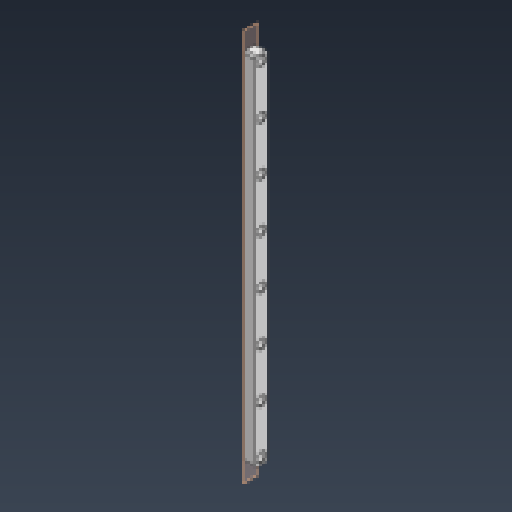
# Autodesk Inventor part: petg_holder
Saved by Autodesk Inventor 2023 (Build 270158000, 158)
## iProperties
Created: 2026-01-24
Part Number: petg_holder
Material: Generic
Document SubType Name: Modeling
Designer: szymo
Density: 1 g/cm^3
Appearance: Default
Author: szymo
Autodesk Inventor part; units mm, degrees
ref_plane "YZ Plane" through (0, 0, 0) normal (1, 0, 0) x (0, 1, 0)
ref_plane "XZ Plane" through (0, 0, 0) normal (0, 1, 0) x (-1, 0, 0)
ref_plane "XY Plane" through (0, 0, 0) normal (0, 0, 1) x (1, 0, 0)
ref_plane "Work Plane1" through (-122.5, -83, 0) normal (1, 0, 0) x (0, -1, 0)
sketch "Sketch1" plane through (-122.5, -83, 0) normal (1, 0, 0) x (0, -1, 0)
  circle A0 centre (-140.1429, -3) radius 1.8 projected
  circle A1 centre (-94.4286, -3) radius 1.8 projected
  circle A2 centre (-48.7143, -3) radius 1.8 projected
  circle A3 centre (-3, -3) radius 1.8 projected
  circle A4 centre (-25.8571, -3) radius 1.8 projected
  circle A5 centre (-71.5714, -3) radius 1.8 projected
  circle A6 centre (-117.2857, -3) radius 1.8 projected
  circle A7 centre (-163, -3) radius 1.8 projected
  line L0 (-166, -6) -> (0, -6) projected
  line L1 (0, 0) -> (0, -6) projected
  line L2 (-166, 0) -> (0, 0) projected
  line L3 (-166, -6) -> (-166, 0) projected
  point P0 (-83, 0)
extrude "Extrusion1" add sketch "Sketch1" along normal blind 5
fillet "Fillet1" radius 1 4 edges at (-120, -83, 0) (-120, -83, 6) (-120, 83, 6) (-120, 83, 0)
sketch "Sketch2" plane through (-117.5, -83, 0) normal (1, 0, 0) x (0, 0, -1)
  arc A0 (0, 165) -> (-1, 166) centre (-1, 165) ccw projected
  line L0 (-1, 166) -> (-5, 166) projected
  arc A1 (-5, 166) -> (-6, 165) centre (-5, 165) ccw projected
  line L1 (-6, 165) -> (-6, 1) projected
  arc A2 (-6, 1) -> (-5, 0) centre (-5, 1) ccw projected
  line L2 (-5, 0) -> (-1, 0) projected
  arc A3 (-1, 0) -> (0, 1) centre (-1, 1) ccw projected
  line L3 (0, 1) -> (0, 165) projected
  circle A4 centre (-3, 163) radius 1.8 projected
  circle A5 centre (-3, 117.2857) radius 1.8 projected
  circle A6 centre (-3, 71.5714) radius 1.8 projected
  circle A7 centre (-3, 25.8571) radius 1.8 projected
  circle A8 centre (-3, 3) radius 1.8 projected
  circle A9 centre (-3, 48.7143) radius 1.8 projected
  circle A10 centre (-3, 94.4286) radius 1.8 projected
  circle A11 centre (-3, 140.1429) radius 1.8 projected
  point P0 (0, 83)
hole "Hole1" at (-117.5, -80, 3) at (-117.5, -57.1429, 3) at (-117.5, -34.2857, 3) at (-117.5, -11.4286, 3) at (-117.5, 11.4286, 3) at (-117.5, 34.2857, 3) at (-117.5, 57.1429, 3) at (-117.5, 80, 3) direction (-1, 0, 0) diameter 4 end through all counterbore diameter 4.5 counterbore depth 0.5
body "Solid1"
